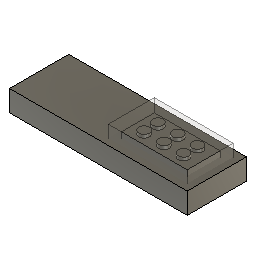
Lego_brick v5 (Autodesk Fusion 360 design; units mm, degrees)
Autodesk Fusion 360 part; units mm, degrees
sketch "Sketch1" plane through (0, 0, 0) normal (0, 0, 1) x (1, 0, 0)
  line L0 (0, 0) -> (100, 0)
  line L1 (100, 0) -> (100, 50)
  line L2 (100, 50) -> (0, 50)
  line L3 (0, 50) -> (0, 0)
  constraint horizontal L0
  constraint vertical L1
  constraint horizontal L2
  constraint vertical L3
  constraint coincident L0.start L3.end
extrude "Extrude1" add sketch "Sketch1" along normal blind 15 and the other way blind 15 makes body 1
sketch "Sketch2" plane through (0, 0, 15) normal (0, 0, 1) x (-1, 0, 0)
  line L0 (0, -50) -> (0, 0)
  line L1 (0, 0) -> (-100, 0)
  line L2 (-100, 0) -> (-100, -50)
  line L3 (-100, -50) -> (0, -50)
  line L4 (0, -50) -> (-5, -50)
  line L5 (-5, -50) -> (-5, -46)
  line L6 (-5, -46) -> (0, -46)
  line L7 (0, -46) -> (0, -50)
  line L8 (-5, -46) -> (-95, -46)
  line L9 (-95, -46) -> (-95, -4)
  line L10 (-95, -4) -> (-5, -4)
  line L11 (-5, -4) -> (-5, -46)
  line L12 (-5, -4) -> (-95, -4)
  line L13 (-95, -4) -> (-95, -25)
  line L14 (-95, -25) -> (-5, -25)
  line L15 (-5, -25) -> (-5, -4)
  line L16 (-5, -4) -> (-35, -4)
  line L17 (-35, -4) -> (-35, -46)
  line L18 (-35, -4) -> (-65, -4)
  line L19 (-65, -4) -> (-65, -46)
  line L20 (-95, -46) -> (-95, -35.5)
  line L21 (-95, -35.5) -> (-80, -35.5)
  circle A0 centre (-80, -35.5) radius 8
  line L22 (-80, -35.5) -> (-20, -35.5)
  line L23 (-20, -35.5) -> (-50, -35.5)
  circle A1 centre (-50, -35.5) radius 8
  circle A2 centre (-20, -35.5) radius 8
  circle A3 centre (-20, -14.5) radius 8
  circle A4 centre (-50, -14.5) radius 8
  circle A5 centre (-80, -14.5) radius 8
  dimension "d5" = 5
  dimension "d6" = 4
  dimension "d7" = 90
  dimension "d8" = 42
  dimension "d9" = 30
  dimension "d10" = 30
  dimension "d11" = 10.5
  dimension "d12" = 16
  dimension "d13" = 16
  dimension "d14" = 16
  constraint perpendicular L4 L5
  constraint parallel L4 L6
  constraint parallel L5 L7
  constraint coincident L3 L4.end
  constraint perpendicular L0 L4
  constraint coincident L0.start L3.end
  constraint perpendicular L8 L9
  constraint parallel L8 L10
  constraint parallel L9 L11
  constraint perpendicular L5 L8
  constraint horizontal L12
  constraint vertical L13
  constraint horizontal L14
  constraint vertical L15
  constraint midpoint L9 L13.end
  constraint perpendicular L15 L16
  constraint coincident L8 L17.end
  constraint perpendicular L8 L17
  constraint perpendicular L17 L18
  constraint coincident L8 L19.end
  constraint perpendicular L8 L19
  constraint perpendicular L8 L20
  constraint perpendicular L20 L21
  constraint coincident L21.end A0.centre
  constraint perpendicular L11 L22
  constraint midpoint L22 L23.end
  constraint coincident L23.end A1.centre
  constraint coincident L22.end L23.start
  constraint symmetric L14 A0 A5
  constraint symmetric L14 A1 A4
  constraint symmetric L14 A2 A3
  measures "d5" distance of L0.start L4.end
  measures "d6" distance of L0.start L6.end
  measures "d7" distance of L5.end L8.end
  measures "d8" distance of L5.end L10.end
  measures "d9" distance of L10.end L16.end
  measures "d10" distance of L16.end L18.end
  measures "d11" distance of L8.end L20.end
  measures "d12" diameter of A0
  measures "d13" diameter of A1
  measures "d14" diameter of A2
extrude "Extrude2" add sketch "Sketch2" along normal blind 5 contours L22 L23 A1 | L22 L23 A1 | L21 A0 L22 | L21 A0 L22 | A2 | A3 | A4 | A5 bodies 1
sketch "Sketch5" plane through (0, 0, 0) normal (0, 0, 1) x (1, 0, 0)
  line L0 (-10, -10) -> (110, -10)
  line L1 (110, -10) -> (110, 60)
  line L2 (110, 60) -> (-10, 60)
  line L3 (-10, 60) -> (-10, -10)
  line L4 (-10, -10) -> (110, 60) construction
  line L5 (110, -10) -> (-10, 60) construction
  point P0 (50, 25)
  dimension "d17" = 120
  dimension "d18" = 70
  constraint horizontal L0
  constraint perpendicular L0 L1
  constraint parallel L0 L2
  constraint parallel L1 L3
  constraint coincident L4 P0
  constraint coincident L5 P0
  measures "d17" distance of L1.end L2.end
  measures "d18" distance of L0.end L1.end
extrude "Extrude3" add sketch "Sketch5" along normal blind 25 and the other way blind 25 separate body makes body 2
combine "Combine1" operation cut target body 2 tool bodies 1 keep tools result as body 3 in component "Lego mold bottom"
ref_plane "WorkPlane1" through (50, 25, 0) normal (0, 0, 1) x (1, 0, 0)
split "Split1" by plane through (50, 25, 0) normal (0, 0, 1) bodies 3 makes body 4 at (30, 36.6667, 25) in component "Lego mold bottom"
box "BoxPrimitive1" add length 5 width 5 height 2 placed x (0, -1, 0) y (1, 0, 0) z (0, 0, 1) at (-7.5, 57.5, 0) bodies 3 in component "Lego mold bottom"
pattern_linear "R-Pattern1" count 2 spacing 110 along (1, 0, 0) count 2 spacing 60 along (0, -1, 0) of "BoxPrimitive1" in component "Lego mold bottom"
combine "Combine1'" operation cut target body 4 tool bodies 3 keep tools result as body 5 in component "Lego mold top"
sketch "Sketch8" plane through (-10, 0, 0) normal (-1, 0, 0) x (0, -1, 0)
  line L0 (10, 0) -> (-60, 0)
  line L1 (-60, 0) -> (-60, -25)
  line L2 (-60, -25) -> (10, -25)
  line L3 (10, -25) -> (10, 0)
  line L4 (-27.5, -2.5) -> (-22.5, -2.5)
  line L5 (-22.5, -2.5) -> (-22.5, 2.5)
  line L6 (-22.5, 2.5) -> (-27.5, 2.5)
  line L7 (-27.5, 2.5) -> (-27.5, -2.5)
  line L8 (-27.5, -2.5) -> (-22.5, 2.5) construction
  line L9 (-22.5, -2.5) -> (-27.5, 2.5) construction
  point P0 (-25, 0)
  dimension "d55" = 5
  dimension "d56" = 5
  constraint horizontal L4
  constraint perpendicular L4 L5
  constraint parallel L4 L6
  constraint parallel L5 L7
  constraint coincident L8 P0
  constraint coincident L9 P0
  constraint midpoint L0 P0
  measures "d55" distance of L5.end L6.end
  measures "d56" distance of L4.end L5.end
extrude "Extrude2'" cut sketch "Sketch8" against normal blind 10 contours L0 L4 L5 L7 | L0 L5 L6 L7 bodies 3 in component "Lego mold bottom"
extrude "Extrude2''" cut sketch "Sketch8" against normal blind 10 contours L0 L4 L5 L7 | L0 L5 L6 L7 bodies 5 in component "Lego mold top"
move_body "Align1" bodies 5 to x (-1, 0, 0) y (0, 1, 0) z (0, 0, -1) at (-20, 0, 0) in component "Lego mold top"
move_body "Move1" bodies 5 to x (1, 0, 0) y (0, 1, 0) z (0, 0, 1) at (-10, 0, 0) in component "Lego mold top"
sketch "Sketch7" plane through (0, 0, 0) normal (0, 0, 1) x (1, 0, 0)
  line L0 (-150, -20) -> (120, -20)
  line L1 (120, -20) -> (120, 70)
  line L2 (120, 70) -> (-150, 70)
  line L3 (-150, 70) -> (-150, -20)
  line L4 (-150, -20) -> (120, 70) construction
  line L5 (120, -20) -> (-150, 70) construction
  point P0 (-15, 25)
  constraint horizontal L0
  constraint perpendicular L0 L1
  constraint parallel L0 L2
  constraint parallel L1 L3
  constraint coincident L4 P0
  constraint coincident L5 P0
extrude "Extrude1'" add sketch "Sketch7" along normal blind 7 and the other way blind 25 separate body makes body 6 in component "Lego mold bottom"
extrude "Extrude1''" [no effect] in component "Lego mold top"
combine "Combine1''" [rolled back] in component "Component"
component "Lego mold bottom" placed x (1, 0, 0) y (0, 1, 0) z (0, 0, 1) at (0, 0, 0)
component "Lego mold top" placed x (1, 0, 0) y (0, 1, 0) z (0, 0, 1) at (0, 0, 0)
component "Component" placed x (1, 0, 0) y (0, 1, 0) z (0, 0, 1) at (0, 0, 0)
hidden bodies 4
named bodies: "Lego", "Mold", "bottom", "top"
